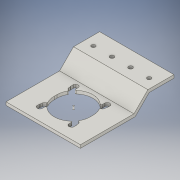
# Autodesk Inventor part: X Motor Mount
Saved by Autodesk Inventor 2019 (Build 230136000, 136)
## iProperties
Created: 2018-01-18
Part Number: X Motor Mount
Material: Steel
Document SubType Name: Modeling
Designer: torba
Density: 7.85 g/cm^3
Appearance: Steel
Author: torba
Autodesk Inventor part; units mm, degrees
ref_plane "YZ Plane" through (0, 0, 0) normal (1, 0, 0) x (0, 1, 0)
ref_plane "XZ Plane" through (0, 0, 0) normal (0, 1, 0) x (-1, 0, 0)
ref_plane "XY Plane" through (0, 0, 0) normal (0, 0, 1) x (1, 0, 0)
sketch "Sketch1" plane through (0, 0, 0) normal (0, 1, 0) x (-1, 0, 0)
  line L0 (25.6794, 50.8) -> (190.2206, 50.8) construction
  line L1 (215.9, 24.892) -> (215.9, 0) construction
  line L2 (215.9, 24.892) -> (196.85, 24.892) construction
  arc A0 (190.2206, 31.5214) -> (196.85, 24.892) centre (196.85, 31.5214) ccw construction
  line L3 (190.2206, 50.8) -> (190.2206, 31.5214) construction
  line L4 (215.9, 0) -> (0, 0) construction
  line L5 (0, 0) -> (0, 24.892) construction
  line L6 (19.05, 24.892) -> (0, 24.892) construction
  arc A1 (19.05, 24.892) -> (25.6794, 31.5214) centre (19.05, 31.5214) ccw construction
  line L7 (25.6794, 31.5214) -> (25.6794, 50.8) construction
  circle A2 centre (50.8, 19.05) radius 3.9687
  circle A3 centre (88.9, 19.05) radius 4.2164
  circle A4 centre (127, 19.05) radius 4.2164
  circle A5 centre (165.1, 19.05) radius 3.9687
  line L8 (190.2206, 50.8) -> (25.6794, 50.8) construction
  line L9 (25.6794, 50.8) -> (25.6794, 0)
  line L10 (25.6794, 0) -> (190.2206, 0)
  line L11 (190.2206, 0) -> (190.2206, 50.8)
  line L12 (190.2206, 50.8) -> (25.6794, 50.8) construction
  line L13 (190.2206, 0) -> (25.6794, 0)
  line L14 (25.6794, 0) -> (25.6794, 127)
  line L15 (25.6794, 127) -> (190.2206, 127)
  line L16 (190.2206, 127) -> (190.2206, 0)
  circle A6 centre (107.4963, 155.5177) radius 2.8
  circle A7 centre (156.7088, 204.7302) radius 2.8
  circle A8 centre (107.4963, 253.9427) radius 2.8
  circle A9 centre (58.2838, 204.7302) radius 2.8
  line L17 (51.4942, 210.0836) -> (102.1428, 260.7323)
  arc A10 (51.4942, 210.0836) -> (51.4942, 199.3767) centre (56.8476, 204.7302) ccw
  line L18 (102.1428, 148.728) -> (51.4942, 199.3767)
  arc A11 (102.1428, 148.728) -> (112.8498, 148.728) centre (107.4963, 154.0815) ccw
  line L19 (163.4984, 199.3767) -> (112.8498, 148.728)
  arc A12 (163.4984, 199.3767) -> (163.4984, 210.0836) centre (158.1449, 204.7302) ccw
  line L20 (112.8498, 260.7323) -> (163.4984, 210.0836)
  arc A13 (112.8498, 260.7323) -> (102.1428, 260.7323) centre (107.4963, 255.3788) ccw
  circle A14 centre (107.4963, 204.7302) radius 36.7665
  point P0 (0, 0)
  point P1 (107.95, 127)
  dimension "d0" = 6.6294
  dimension "d1" = 7.9375
  dimension "d2" = 8.4328
  dimension "d3" = 90
  dimension "d4" = 25.6794
  dimension "d5" = 190.2206
  dimension "d6" = 215.9
  dimension "d7" = 50.8
  dimension "d8" = 24.892
  dimension "d9" = 24.892
  dimension "d10" = 215.9
  dimension "d11" = 0
  dimension "d12" = 5.842
  dimension "d13" = 50.8
  dimension "d14" = 5.842
  dimension "d15" = 88.9
  dimension "d16" = 5.842
  dimension "d17" = 127
  dimension "d18" = 5.842
  dimension "d19" = 165.1
  dimension "d20" = 50.8
  dimension "d22" = 127
  dimension "d23" = 190.2206
  dimension "d24" = 190.2206
  constraints: 42 end point, 15 centre point, 12 point on circle, 9 parallel, 5 tangent, 4 horizontal, 3 equal radius, 2 perpendicular, 1 midpoint, 1 point on line, 1 vertical
  measures "d0" radius of A0
  measures "d1" diameter of A5
  measures "d2" diameter of A4
  measures "d3" angle of L2 L1
  measures "d4" distance between parallel lines of L1 L3
  measures "d5" distance between parallel lines of L1 L7
  measures "d6" distance between parallel lines of L1 L5
  measures "d7" distance between parallel lines of L4 L0
  measures "d8" distance between parallel lines of L4 L6
  measures "d9" distance from line of point (0, 0) L2
  measures "d10" distance from line of point (0, 0) L1
  measures "d11" distance from line of point (0, 0) L4
  measures "d12" distance from line of A5.centre L2
  measures "d13" distance from line of A5.centre L1
  measures "d14" distance from line of A4.centre L2
  measures "d15" distance from line of A4.centre L1
  measures "d16" distance from line of A3.centre L2
  measures "d17" distance from line of A3.centre L1
  measures "d18" distance from line of A2.centre L2
  measures "d19" distance from line of A2.centre L1
  measures "d20" distance from line of L5 A2.centre
  measures "d22" distance of L13.end L14.end
  measures "d23" distance between parallel lines of L9 L1
  measures "d24" distance from line of L12.end L1
extrude "Extrusion1" add sketch "Sketch1" along normal blind 6.35 contours L14 L15 L16 L11 L10 L9
sketch "Sketch2" plane through (0, 6.35, 0) normal (0, 1, 0) x (1, 0, 0)
  circle A0 centre (-88.9, -19.05) radius 4.2164 construction
  circle A1 centre (-127, -19.05) radius 4.2164 construction
  circle A2 centre (-50.8, -19.05) radius 3.9687 construction
  circle A3 centre (-165.1, -19.05) radius 3.9687 construction
  line L0 (-25.6794, 0) -> (-190.2206, 0) construction
  line L1 (-190.2206, 0) -> (-190.2206, -127) construction
  line L2 (-190.2206, -127) -> (-25.6794, -127) construction
  line L3 (-25.6794, -127) -> (-25.6794, 0) construction
  circle A4 centre (-168.9341, -105.7135) radius 2.8
  circle A5 centre (-99.3372, -105.7135) radius 2.8
  circle A6 centre (-99.3372, -36.1166) radius 2.8
  circle A7 centre (-168.9341, -36.1166) radius 2.8
  line L4 (-169.9497, -27.5301) -> (-98.3217, -27.5301) construction
  arc A8 (-169.9497, -27.5301) -> (-177.5206, -35.1011) centre (-169.9497, -35.1011) ccw construction
  line L5 (-177.5206, -106.7291) -> (-177.5206, -35.1011) construction
  arc A9 (-177.5206, -106.7291) -> (-169.9497, -114.3) centre (-169.9497, -106.7291) ccw construction
  line L6 (-98.3217, -114.3) -> (-169.9497, -114.3) construction
  arc A10 (-98.3217, -114.3) -> (-90.7507, -106.7291) centre (-98.3217, -106.7291) ccw construction
  line L7 (-90.7507, -35.1011) -> (-90.7507, -106.7291) construction
  arc A11 (-90.7507, -35.1011) -> (-98.3217, -27.5301) centre (-98.3217, -35.1011) ccw construction
  circle A12 centre (-134.1357, -70.9151) radius 36.7665
  line L8 (-134.1357, -70.9151) -> (-177.5206, -70.9151) construction
  line L9 (-177.5206, -70.9151) -> (-177.5206, -114.3) construction
  line L10 (-177.5206, -114.3) -> (-134.1357, -114.3) construction
  line L11 (-134.1357, -114.3) -> (-134.1357, -70.9151) construction
  line L12 (-134.1357, -70.9151) -> (-177.5206, -70.9151) construction
  line L13 (-177.5206, -70.9151) -> (-177.5206, -27.5301) construction
  line L14 (-177.5206, -27.5301) -> (-134.1357, -27.5301) construction
  line L15 (-134.1357, -27.5301) -> (-134.1357, -70.9151) construction
  line L16 (-134.1357, -70.9151) -> (-90.7507, -70.9151) construction
  line L17 (-90.7507, -70.9151) -> (-90.7507, -27.5301) construction
  line L18 (-90.7507, -27.5301) -> (-134.1357, -27.5301) construction
  line L19 (-134.1357, -27.5301) -> (-134.1357, -70.9151) construction
  line L20 (-134.1357, -70.9151) -> (-90.7507, -70.9151) construction
  line L21 (-90.7507, -70.9151) -> (-90.7507, -114.3) construction
  line L22 (-90.7507, -114.3) -> (-134.1357, -114.3) construction
  line L23 (-134.1357, -114.3) -> (-134.1357, -70.9151) construction
  line L24 (-190.2206, 0) -> (-190.2206, -127) construction
  line L25 (-25.6794, 0) -> (-190.2206, 0) construction
  line L26 (-190.2206, -127) -> (-183.8706, -127) construction
  line L27 (-183.8706, -127) -> (-183.8706, 0) construction
  line L28 (-183.8706, 0) -> (-190.2206, 0) construction
  line L29 (-190.2206, 0) -> (-190.2206, -127) construction
  line L30 (-190.2206, -127) -> (-25.6794, -127) construction
  line L31 (-25.6794, -127) -> (-32.0294, -127) construction
  line L32 (-32.0294, -127) -> (-32.0294, 0) construction
  line L33 (-32.0294, 0) -> (-25.6794, 0) construction
  line L34 (-25.6794, 0) -> (-25.6794, -127) construction
  line L35 (-25.6794, -127) -> (-25.6794, 0) construction
  line L36 (-190.2206, -127) -> (-25.6794, -127) construction
  line L37 (-25.6794, -127) -> (-25.6794, -120.65) construction
  line L38 (-25.6794, -120.65) -> (-190.2206, -120.65) construction
  line L39 (-190.2206, -120.65) -> (-190.2206, -127) construction
  line L40 (-183.8706, -120.65) -> (-177.5206, -120.65) construction
  line L41 (-177.5206, -120.65) -> (-177.5206, -114.3) construction
  line L42 (-177.5206, -114.3) -> (-183.8706, -114.3) construction
  line L43 (-183.8706, -114.3) -> (-183.8706, -120.65) construction
  point P0 (0, 0)
  constraints: 72 end point, 16 parallel, 9 centre point, 9 point on line, 8 horizontal, 8 perpendicular, 8 point on circle, 8 tangent, 6 equal radius
sketch "Sketch3" plane through (0, 6.35, 0) normal (0, 1, 0) x (1, 0, 0)
  circle A0 centre (-88.9, -19.05) radius 4.2164 projected
  circle A1 centre (-127, -19.05) radius 4.2164 projected
  circle A2 centre (-50.8, -19.05) radius 3.9687 projected
  circle A3 centre (-165.1, -19.05) radius 3.9687 projected
  line L0 (-25.6794, 0) -> (-190.2206, 0) projected
  line L1 (-190.2206, 0) -> (-190.2206, -127) projected
  line L2 (-190.2206, -127) -> (-25.6794, -127) projected
  line L3 (-25.6794, -127) -> (-25.6794, 0) projected
  point P0 (0, 0)
extrude "Extrusion3" add sketch "Sketch3" against normal up to surface (6.35 mm away) contours A0 | A1 | A2 | A3
sketch "Sketch5" plane through (0, 6.35, 0) normal (0, 1, 0) x (1, 0, 0)
  line L0 (-25.6794, 0) -> (-190.2206, 0) projected
  line L1 (-190.2206, 0) -> (-190.2206, -127) projected
  line L2 (-190.2206, -127) -> (-25.6794, -127) projected
  line L3 (-25.6794, -127) -> (-25.6794, 0) projected
  line L4 (-190.2206, -127) -> (-25.6794, -127)
  line L5 (-25.6794, -127) -> (-25.6794, -138.176)
  line L6 (-25.6794, -138.176) -> (-190.2206, -138.176)
  line L7 (-190.2206, -138.176) -> (-190.2206, -127)
  line L8 (-134.1357, -70.9151) -> (-134.1357, -3.6559)
  line L9 (-190.2206, -127) -> (-190.2206, 0) projected
  line L10 (-25.6794, 0) -> (-25.6794, -127) projected
  line L11 (-190.2206, 0) -> (-25.6794, 0)
  line L12 (-25.6794, 0) -> (-25.6794, -3.6559)
  line L13 (-25.6794, -3.6559) -> (-190.2206, -3.6559)
  line L14 (-190.2206, -3.6559) -> (-190.2206, 0)
  point P0 (0, 0)
  dimension "d61" = 11.176
  dimension "d62" = 67.2592
  constraints: 18 end point, 4 parallel, 3 perpendicular, 2 horizontal, 1 point on line
  measures "d61" distance of L4.end L5.end
  measures "d62" distance of L8.start L8.end
extrude "Extrusion4" add sketch "Sketch5" against normal up to surface (6.35 mm away) contours L5 L6 L7 L2
sketch "Sketch6" plane through (-190.2206, 6.35, 138.176) normal (0, 0, 1) x (1, 0, 0)
  line L0 (164.5412, -6.35) -> (0, -6.35) projected
  line L1 (164.5412, 0) -> (164.5412, -6.35) projected
  line L2 (0, 0) -> (164.5412, 0) projected
  line L3 (0, 0) -> (0, -6.35) projected
  point P0 (190.2206, -6.35)
extrude "Extrusion5" add sketch "Sketch6" along normal blind 12.7
sketch "Sketch7" plane through (-25.6794, 0, 0) normal (0, 0, -1) x (-1, 0, 0)
  line L0 (164.5412, 0) -> (0, 0) projected
  line L1 (164.5412, 0) -> (164.5412, 6.35) projected
  line L2 (0, 6.35) -> (164.5412, 6.35) projected
  line L3 (0, 0) -> (0, 6.35) projected
  point P0 (-25.6794, 0)
extrude "Extrusion6" add sketch "Sketch7" along normal blind 7.874
sketch "Sketch9" plane through (-190.2206, 0, 150.876) normal (-1, 0, 0) x (0, 0, 1)
  line L0 (0, 6.35) -> (-158.75, 6.35) projected
  line L1 (-158.75, 6.35) -> (-130.175, 6.35)
  line L2 (-130.175, 6.35) -> (-130.175, 0)
  line L3 (0, 0) -> (-158.75, 0) projected
  line L4 (-130.175, 0) -> (-158.75, 28.575)
  line L5 (-130.175, 0) -> (-89.7638, 0) construction
  line L6 (-158.75, 28.575) -> (-154.2599, 33.0651)
  line L7 (-158.75, 28.575) -> (-152.4, 28.575) construction
  line L8 (-154.2599, 33.0651) -> (-127.5447, 6.35)
  line L9 (-158.75, 28.575) -> (-209.55, 28.575)
  line L10 (-209.55, 28.575) -> (-209.55, 34.925)
  line L11 (-209.55, 34.925) -> (-156.1197, 34.925)
  line L12 (-154.2599, 33.0651) -> (-156.1197, 34.925)
  point P0 (-150.876, 0)
  dimension "d69" = 28.575
  dimension "d70" = 135
  dimension "d71" = 6.35
  dimension "d72" = 45
  dimension "d73" = 50.8
  dimension "d74" = 6.35
  dimension "d75" = 135
  dimension "d76" = 28.575
  constraints: 22 end point, 3 horizontal, 3 perpendicular, 3 point on line, 2 equal length, 1 vertical
  measures "d69" distance of L0.end L1.end
  measures "d70" angle of L5 L4
  measures "d71" distance of L4.end L6.end
  measures "d72" angle of L7 L6
  measures "d73" distance of L4.end L9.end
  measures "d74" distance of L9.end L10.end
  measures "d75" angle of L12 L0
  measures "d76" distance between parallel lines of L11 L0
extrude "Extrusion7" add sketch "Sketch9" against normal up to surface (164.5412 mm away)
sketch "Sketch11" plane through (-190.2206, 0, 150.876) normal (-1, 0, 0) x (0, 0, 1)
  line L0 (-136.525, 6.35) -> (-158.75, 6.35) projected
  line L1 (-158.75, 0) -> (-158.75, 6.35) projected
  line L2 (0, 0) -> (-158.75, 0) projected
  line L3 (0, 6.35) -> (0, 0) projected
  line L4 (0, 6.35) -> (-127.5447, 6.35) projected
  line L5 (-127.5447, 6.35) -> (-156.1197, 34.925) projected
  line L6 (-156.1197, 34.925) -> (-209.55, 34.925) projected
  line L7 (-209.55, 34.925) -> (-209.55, 28.575) projected
  line L8 (-209.55, 28.575) -> (-158.75, 28.575) projected
  line L9 (-158.75, 28.575) -> (-136.525, 6.35) projected
  line L10 (0, 0) -> (-158.75, 0) projected
  line L11 (-158.75, 6.35) -> (-136.525, 6.35)
  line L12 (-136.525, 6.35) -> (-136.525, 0) construction
  line L13 (-136.525, 0) -> (-158.75, 0)
  line L14 (-158.75, 0) -> (-158.75, 6.35)
  line L15 (-136.525, 6.35) -> (-130.175, 0)
  line L16 (-130.175, 0) -> (-136.525, 0)
  point P0 (-150.876, 0)
  constraints: 12 end point, 3 point on line, 2 parallel, 1 collinear, 1 horizontal, 1 perpendicular
extrude "Extrusion9" cut sketch "Sketch11" against normal through all contours L15 L2 L1 L0
sketch "Sketch12" plane through (-25.6794, 0, 150.876) normal (1, 0, 0) x (0, 0, -1)
  line L0 (130.175, 0) -> (158.75, 28.575) projected
  line L1 (209.55, 28.575) -> (158.75, 28.575) projected
  line L2 (209.55, 34.925) -> (209.55, 28.575) projected
  line L3 (156.1197, 34.925) -> (209.55, 34.925) projected
  line L4 (127.5447, 6.35) -> (156.1197, 34.925) projected
  line L5 (0, 6.35) -> (127.5447, 6.35) projected
  line L6 (0, 0) -> (0, 6.35) projected
  line L7 (130.175, 0) -> (0, 0) projected
  point P0 (150.876, 0)
extrude "Extrusion10" cut sketch "Sketch12" against normal blind 12.1412
sketch "Sketch13" plane through (0, 6.35, 0) normal (0, 1, 0) x (1, 0, 0)
  line L0 (-37.8206, -150.876) -> (-37.8206, -23.3313) projected
  line L1 (-37.8206, -23.3313) -> (-190.2206, -23.3313) projected
  line L2 (-190.2206, -150.876) -> (-190.2206, -23.3313) projected
  line L3 (-37.8206, -150.876) -> (-190.2206, -150.876) projected
  line L4 (-37.8206, -20.701) -> (-37.8206, -150.876) projected
  line L5 (-190.2206, -150.876) -> (-190.2206, -20.701) projected
  line L6 (-190.2206, -150.876) -> (-190.2206, -70.9151)
  line L7 (-190.2206, -70.9151) -> (-37.8206, -70.9151) construction
  line L8 (-37.8206, -150.876) -> (-37.8206, -23.3313) projected
  line L9 (-148.8191, -33.3166) -> (-148.8191, -38.9166) construction
  line L10 (-79.2221, -33.3166) -> (-79.2221, -38.9166) construction
  line L11 (-79.2221, -102.9135) -> (-79.2221, -108.5135) construction
  line L12 (-148.8191, -102.9135) -> (-148.8191, -108.5135) construction
  line L13 (-114.0206, -70.9151) -> (-114.0206, -68.1211)
  line L14 (-114.0206, -68.1211) -> (-114.0206, -73.7091)
  line L15 (-148.8191, -33.3166) -> (-148.8191, -38.9166) construction
  line L16 (-151.6191, -33.3166) -> (-151.6191, -38.9166)
  line L17 (-146.0191, -38.9166) -> (-146.0191, -33.3166)
  arc A0 (-146.0191, -33.3166) -> (-151.6191, -33.3166) centre (-148.8191, -33.3166) ccw
  arc A1 (-151.6191, -38.9166) -> (-146.0191, -38.9166) centre (-148.8191, -38.9166) ccw
  line L18 (-148.8191, -102.9135) -> (-148.8191, -108.5135) construction
  line L19 (-151.6191, -102.9135) -> (-151.6191, -108.5135)
  line L20 (-146.0191, -108.5135) -> (-146.0191, -102.9135)
  arc A2 (-146.0191, -102.9135) -> (-151.6191, -102.9135) centre (-148.8191, -102.9135) ccw
  arc A3 (-151.6191, -108.5135) -> (-146.0191, -108.5135) centre (-148.8191, -108.5135) ccw
  line L21 (-114.0206, -68.1211) -> (-114.0206, -73.7091) construction
  line L22 (-150.7871, -68.1211) -> (-150.7871, -73.7091)
  line L23 (-77.2541, -73.7091) -> (-77.2541, -68.1211)
  arc A4 (-77.2541, -68.1211) -> (-150.7871, -68.1211) centre (-114.0206, -68.1211) ccw
  arc A5 (-150.7871, -73.7091) -> (-77.2541, -73.7091) centre (-114.0206, -73.7091) ccw
  line L24 (-79.2221, -33.3166) -> (-79.2221, -38.9166) construction
  line L25 (-82.0221, -33.3166) -> (-82.0221, -38.9166)
  line L26 (-76.4221, -38.9166) -> (-76.4221, -33.3166)
  arc A6 (-76.4221, -33.3166) -> (-82.0221, -33.3166) centre (-79.2221, -33.3166) ccw
  arc A7 (-82.0221, -38.9166) -> (-76.4221, -38.9166) centre (-79.2221, -38.9166) ccw
  line L27 (-79.2221, -102.9135) -> (-79.2221, -108.5135) construction
  line L28 (-82.0221, -102.9135) -> (-82.0221, -108.5135)
  line L29 (-76.4221, -108.5135) -> (-76.4221, -102.9135)
  arc A8 (-76.4221, -102.9135) -> (-82.0221, -102.9135) centre (-79.2221, -102.9135) ccw
  arc A9 (-82.0221, -108.5135) -> (-76.4221, -108.5135) centre (-79.2221, -108.5135) ccw
  circle A10 centre (-148.8191, -36.1166) radius 1.27
  circle A11 centre (-79.2221, -36.1166) radius 1.27
  circle A12 centre (-79.2221, -105.7135) radius 1.27
  circle A13 centre (-114.0206, -70.9151) radius 1.27
  circle A14 centre (-148.8191, -105.7135) radius 1.27
  point P0 (0, 0)
  dimension "d87" = 47.5838
  dimension "d117" = 5.588
  dimension "d118" = 2.54
  dimension "d119" = 2.54
  dimension "d120" = 2.54
  dimension "d121" = 2.54
  dimension "d122" = 2.54
  dimension "d123" = 2.8
  dimension "d124" = 2.8
  dimension "d125" = 36.7665
  dimension "d126" = 38.6015
  dimension "d127" = 110.9985
  dimension "d128" = 79.5823
  dimension "d129" = 44.7898
  dimension "d130" = 117.5594
  dimension "d131" = 9.9853
  dimension "d132" = 79.5823
  constraints: 56 end point, 26 tangent, 20 point on circle, 15 centre point, 10 parallel, 7 point on line, 6 midpoint, 5 coincident, 2 collinear, 1 equal radius, 1 perpendicular, 1 vertical
  measures "d87" distance between parallel lines of L1 L7
  measures "d117" distance of L13.end L14.end
  measures "d118" diameter of A10
  measures "d119" diameter of A11
  measures "d120" diameter of A12
  measures "d121" diameter of A13
  measures "d122" diameter of A14
  measures "d123" radius of A6
  measures "d124" radius of A8
  measures "d125" radius of A4
  measures "d126" distance between parallel lines of L0 L26
  measures "d127" distance between parallel lines of L0 L9
  measures "d128" distance from line of L29.end L1
  measures "d129" distance from line of L23.end L1
  measures "d130" distance from line of L10.start L3
  measures "d131" distance from line of L17.end L1
  measures "d132" distance from line of L20.end L1
sketch "Sketch14" plane through (0, 6.35, 0) normal (0, 1, 0) x (1, 0, 0)
  circle A0 centre (-114.0206, -70.9151) radius 36.7665 projected
  line L0 (-37.8206, -150.876) -> (-37.8206, -23.3313) projected
  line L1 (-37.8206, -23.3313) -> (-190.2206, -23.3313) projected
  line L2 (-190.2206, -150.876) -> (-190.2206, -23.3313) projected
  line L3 (-37.8206, -150.876) -> (-190.2206, -150.876) projected
  line L4 (-114.0206, -70.9151) -> (-114.0206, -118.4893)
  line L5 (-114.0206, -107.6816) -> (-114.0206, -133.0816)
  line L6 (-37.8206, -150.876) -> (-37.8206, -23.3313) projected
  line L7 (-190.2206, -150.876) -> (-190.2206, -20.701) projected
  line L8 (-37.8206, -150.876) -> (-190.2206, -150.876)
  line L9 (-190.2206, -150.876) -> (-190.2206, -133.0816)
  line L10 (-190.2206, -133.0816) -> (-37.8206, -133.0816)
  line L11 (-37.8206, -133.0816) -> (-37.8206, -150.876)
  point P0 (0, 0)
  dimension "d100" = 47.5742
  dimension "d101" = 25.4
  dimension "d104" = 17.7945
  constraints: 12 end point, 3 point on line, 2 parallel, 1 horizontal, 1 perpendicular, 1 vertical
  measures "d100" distance of L4.start L4.end
  measures "d101" distance of L5.start L5.end
  measures "d104" distance between parallel lines of L3 L10
extrude "Extrusion12" cut sketch "Sketch14" against normal through all contours L3 L2 L10 L0
sketch "Sketch15" plane through (-190.2206, 34.925, -5.2437) normal (0, 1, 0) x (1, 0, 0)
  circle A0 centre (19.05, 21.682) radius 3.9687
  circle A1 centre (57.15, 21.682) radius 4.2164
  circle A2 centre (95.25, 21.682) radius 4.2164
  circle A3 centre (133.35, 21.682) radius 3.9687
  point P0 (190.2206, -5.2437)
  dimension "d105" = 7.9375
  dimension "d106" = 8.4328
  dimension "d107" = 62.9227
  dimension "d108" = 98.7138
  dimension "d109" = 135.7674
  dimension "d110" = 173.2754
  dimension "d111" = 38.1
  dimension "d112" = 76.2
  dimension "d113" = 114.3
  constraints: 4 centre point, 2 equal radius
  measures "d105" diameter of A3
  measures "d106" diameter of A2
  measures "d107" distance of point (190.221, -5.244) A3.centre
  measures "d108" distance of point (190.221, -5.244) A2.centre
  measures "d109" distance of point (190.221, -5.244) A1.centre
  measures "d110" distance of point (190.221, -5.244) A0.centre
  measures "d111" distance of A3.centre A2.centre
  measures "d112" distance of A3.centre A1.centre
  measures "d113" distance of A3.centre A0.centre
extrude "Extrusion13" cut sketch "Sketch15" against normal blind 12.1412
extrude "Extrusion14" cut sketch "Sketch13" against normal through all contours A0 L17 A1 L16 | A2 L20 A3 L19 | A4 L23 A5 L22 | A6 L26 A7 L25 | A8 L29 A9 L28
sketch "Sketch18" plane through (0, 0, 0) normal (0, -1, 0) x (1, 0, 0)
  arc A0 (-146.1675, 43.5307) -> (-146.1675, 34.0057) centre (-146.1675, 38.7682) ccw construction
  circle A1 centre (-114.0206, 70.9151) radius 1.27 projected
  circle A2 centre (-114.0206, 70.9151) radius 1.27 projected
  line L0 (-81.8737, 107.8244) -> (-81.8737, 98.2994) construction
  line L1 (-81.8737, 43.5307) -> (-81.8737, 34.0057) construction
  line L2 (-114.8547, 71.8727) -> (-113.1865, 69.9574) construction
  line L3 (-113.1865, 71.8727) -> (-114.8547, 69.9574) construction
  line L4 (-146.1675, 34.0057) -> (-146.1675, 43.5307) construction
  line L5 (-146.1675, 98.2994) -> (-146.1675, 107.8244) construction
  circle A3 centre (-81.8737, 103.0619) radius 4.7625 construction
  line L6 (-82.0221, 33.3166) -> (-82.0221, 38.9166) projected
  circle A4 centre (-146.1675, 103.0619) radius 4.7625 construction
  circle A5 centre (-146.1675, 38.7682) radius 4.7625 construction
  line L7 (-81.8737, 107.8244) -> (-81.8737, 98.2994) construction
  line L8 (-86.6362, 107.8244) -> (-86.6362, 98.2994)
  line L9 (-77.1112, 98.2994) -> (-77.1112, 107.8244)
  arc A6 (-77.1112, 107.8244) -> (-86.6362, 107.8244) centre (-81.8737, 107.8244) ccw
  arc A7 (-86.6362, 98.2994) -> (-77.1112, 98.2994) centre (-81.8737, 98.2994) ccw
  line L10 (-146.1675, 43.5307) -> (-146.1675, 34.0057) construction
  line L11 (-150.93, 43.5307) -> (-150.93, 34.0057)
  line L12 (-141.405, 34.0057) -> (-141.405, 43.5307)
  arc A8 (-141.405, 43.5307) -> (-150.93, 43.5307) centre (-146.1675, 43.5307) ccw
  arc A9 (-150.93, 34.0057) -> (-141.405, 34.0057) centre (-146.1675, 34.0057) ccw
  line L13 (-146.1675, 107.8244) -> (-146.1675, 98.2994) construction
  line L14 (-150.93, 107.8244) -> (-150.93, 98.2994)
  line L15 (-141.405, 98.2994) -> (-141.405, 107.8244)
  arc A10 (-141.405, 107.8244) -> (-150.93, 107.8244) centre (-146.1675, 107.8244) ccw
  arc A11 (-150.93, 98.2994) -> (-141.405, 98.2994) centre (-146.1675, 98.2994) ccw
  circle A12 centre (-81.8737, 38.7682) radius 4.7625 construction
  line L16 (-81.8737, 43.5307) -> (-81.8737, 34.0057) construction
  line L17 (-86.6362, 43.5307) -> (-86.6362, 34.0057)
  line L18 (-77.1112, 34.0057) -> (-77.1112, 43.5307)
  arc A13 (-77.1112, 43.5307) -> (-86.6362, 43.5307) centre (-81.8737, 43.5307) ccw
  arc A14 (-86.6362, 34.0057) -> (-77.1112, 34.0057) centre (-81.8737, 34.0057) ccw
  point P0 (-146.1675, 38.7682)
  dimension "d137" = 4.7625
  dimension "d138" = 41.055
  dimension "d139" = 41.055
  dimension "d140" = 0.1484
  dimension "d141" = 64.1454
  dimension "d142" = 52.074
  dimension "d143" = 9.8471
  dimension "d144" = 3.5913
  dimension "d145" = 38.6356
  constraints: 44 end point, 22 point on circle, 20 tangent, 11 equal length, 9 centre point, 9 midpoint, 6 vertical, 4 vertical alignment, 1 coincident, 1 equal radius, 8 other
  measures "d137" radius of A6
  measures "d138" angle of L6 L2
  measures "d139" angle of L6 L3
  measures "d140" distance between parallel lines of L6 L0
  measures "d141" distance between parallel lines of L6 L13
  measures "d142" distance from line of L9.end L2
  measures "d143" distance from line of L18.end L2
  measures "d144" distance from line of L15.end L2
  measures "d145" distance from line of L12.end L2
extrude "Extrusion15" cut sketch "Sketch18" against normal blind 25.4 contours A6 L9 A7 L8 | A8 L12 A9 L11 | A10 L15 A11 L14 | A13 L18 A14 L17
fillet "Fillet1" radius 1.5875 8 edges at (-83.1758, 3.175, 93.7184) (-83.1758, 3.175, 48.1117) (-86.6359, 3.175, 43.5884) (-141.4053, 3.175, 98.2417) (-144.8654, 3.175, 93.7184) (-141.4053, 3.175, 43.5884) (-144.8654, 3.175, 48.1117) (-86.6359, 3.175, 98.2417)
body "Solid1"
